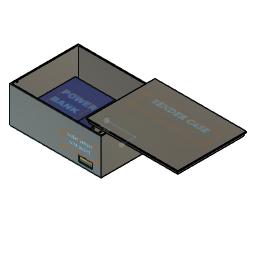
Sender case (Autodesk Fusion 360 design; units mm, degrees)
part number: 2025-07-08-07-24-11-456
Autodesk Fusion 360 part; units mm, degrees
sketch "Sketch1" plane through (0, 0, 0) normal (0, 0, 1) x (1, 0, 0)
  line L0 (80, -60) -> (-80, -60)
  line L1 (-80, -60) -> (-80, 60)
  line L2 (-80, 60) -> (80, 60)
  line L3 (80, 60) -> (80, -60)
  line L4 (80, -60) -> (-80, 60) construction
  line L5 (-80, -60) -> (80, 60) construction
  dimension "d1" = 160
  dimension "d2" = 120
  constraint horizontal L0
  constraint perpendicular L0 L1
  constraint parallel L0 L2
  constraint parallel L1 L3
  constraint coincident L4 origin
  constraint coincident L5 origin
  measures "d1" distance of L1.end L2.end
  measures "d2" distance of L0.end L1.end
extrude "Extrude1" add sketch "Sketch1" along normal blind 35 makes body 1
shell "Shell1" thickness 2 removed faces 1 at (26.6667, -20, 35) on bodies 1
sketch "Sketch2" plane through (0, 0, 35) normal (0, 0, 1) x (-1, 0, 0)
  line L0 (-78, -58) -> (-78, 58)
  line L1 (-78, 58) -> (78, 58)
  line L2 (78, 58) -> (78, -58)
  line L3 (78, -58) -> (-78, -58)
  line L4 (-80, -60) -> (80, -60)
  line L5 (80, -60) -> (80, 60)
  line L6 (80, 60) -> (-80, 60)
  line L7 (-80, 60) -> (-80, -60)
  line L8 (-80, -60) -> (80, -60)
  line L9 (80, -60) -> (80, 60)
extrude "Extrude2" add sketch "Sketch2" along normal blind 7 bodies 1
sketch "Sketch3" plane through (0, 0, 42) normal (0, 0, 1) x (-1, 0, 0)
  line L0 (78, 58) -> (78, -58)
  line L1 (78, -58) -> (-78, -58)
  line L2 (-78, -58) -> (-78, 58)
  line L3 (-78, 58) -> (78, 58)
  line L4 (80, -60) -> (80, 60)
  line L5 (80, 60) -> (-80, 60)
  line L6 (-80, 60) -> (-80, -60)
  line L7 (-80, -60) -> (80, -60)
extrude "Extrude3" add sketch "Sketch3" along normal blind 7 bodies 1
sketch "Sketch4" plane through (0, 0, 0) normal (0, 0, 1) x (1, 0, 0)
  line L0 (80, 60) -> (-80, 60)
  line L1 (-80, 60) -> (-80, -60)
  line L2 (-80, -60) -> (80, -60)
  line L3 (80, -60) -> (80, 60)
  line L4 (80, 60) -> (-80, -60) construction
  line L5 (-80, 60) -> (80, -60) construction
  dimension "d10" = 160
  dimension "d11" = 120
  constraint horizontal L0
  constraint perpendicular L0 L1
  constraint parallel L0 L2
  constraint parallel L1 L3
  constraint coincident L4 origin
  constraint coincident L5 origin
  measures "d10" distance of L1.end L2.end
  measures "d11" distance of L0.end L1.end
extrude "Extrude4" add sketch "Sketch4" along normal blind 7 separate body makes body 2
move_body "Move1" bodies 2 to x (1, 0, 0) y (0, 1, 0) z (0, 0, 1) at (0, 0, 40)
sketch "Sketch5" plane through (0, 0, 49) normal (0, 0, 1) x (-1, 0, 0)
  line L0 (-78, -58) -> (-78, 58)
  line L1 (-78, 58) -> (78, 58)
  line L2 (78, 58) -> (78, -58)
  line L3 (78, -58) -> (-78, -58)
  line L4 (-80, -60) -> (80, -60)
  line L5 (80, -60) -> (80, 60)
  line L6 (80, 60) -> (-80, 60)
  line L7 (-80, 60) -> (-80, -60)
extrude "Extrude5" add sketch "Sketch5" along normal blind 7 bodies 1
sketch "Sketch6" plane through (0, 0, 56) normal (0, 0, 1) x (-1, 0, 0)
  line L0 (78, 58) -> (78, -58)
  line L1 (78, -58) -> (-78, -58)
  line L2 (-78, -58) -> (-78, 58)
  line L3 (-78, 58) -> (78, 58)
  line L4 (-80, 60) -> (-80, -60)
  line L5 (-80, -60) -> (80, -60)
  line L6 (80, -60) -> (80, 60)
  line L7 (80, 60) -> (-80, 60)
  line L8 (-80, 60) -> (-80, -60)
  line L9 (80, 60) -> (-80, 60)
  line L10 (80, -60) -> (80, 60)
  line L11 (-80, -60) -> (80, -60)
extrude "Extrude6" add sketch "Sketch6" along normal blind 7 bodies 1
move_body "Move2" bodies 2 to x (1, 0, 0) y (0, 1, 0) z (0, 0, 1) at (-5.0948, 10.5251, 18.3046)
sketch "Sketch7" plane through (0, 0, 65.3046) normal (0, 0, 1) x (-1, 0, 0)
  line L0 (-74.9052, 49.4749) -> (-74.9052, -70.5251)
  line L1 (-74.9052, -70.5251) -> (85.0948, -70.5251)
  line L2 (85.0948, -70.5251) -> (85.0948, 49.4749)
  line L3 (85.0948, 49.4749) -> (-74.9052, 49.4749)
  line L4 (-74.9052, 49.4749) -> (-74.9052, -70.5251)
  line L5 (-74.9052, -70.5251) -> (85.0948, -70.5251)
  line L6 (85.0948, -70.5251) -> (85.0948, 49.4749)
  line L7 (85.0948, 49.4749) -> (-74.9052, 49.4749)
  line L8 (83.0948, -68.5251) -> (83.0948, 47.4749)
  line L9 (83.0948, 47.4749) -> (-72.9052, 47.4749)
  line L10 (-72.9052, 47.4749) -> (-72.9052, -68.5251)
  line L11 (-72.9052, -68.5251) -> (83.0948, -68.5251)
  dimension "d18" = -2
extrude "Extrude7" cut sketch "Sketch7" against normal blind 5 bodies 1 2
move_body "Move3" bodies 2 to x (1, 0, 0) y (0, 1, 0) z (0, 0, 1) at (0, -11, 0)
move_body "Move4" bodies 2 to x (1, 0, 0) y (0, -1, 0) z (0, 0, -1) at (140, -0.9498, 136.6091)
sketch "Sketch8" plane through (0, 0, 2) normal (0, 0, 1) x (-1, 0, 0)
  line L0 (-78, -58) -> (78, -58)
  line L1 (78, -58) -> (78, 58)
  line L2 (78, 58) -> (-78, 58)
  line L3 (-78, 58) -> (-78, -58)
  line L4 (181.9666, -46.9466) -> (111.9666, -46.9466)
  line L5 (111.9666, -46.9466) -> (111.9666, 53.0534)
  line L6 (111.9666, 53.0534) -> (181.9666, 53.0534)
  line L7 (181.9666, 53.0534) -> (181.9666, -46.9466)
  dimension "d21" = 70
  dimension "d22" = 100
  constraint horizontal L4
  constraint vertical L5
  constraint horizontal L6
  constraint vertical L7
  measures "d21" distance of L4.start L4.end
  measures "d22" distance of L4.start L6.end
extrude "Extrude8" add sketch "Sketch8" along normal blind 22 separate body contours L4 L5 L6 L7 makes body 3
move_body "Move5" bodies 3 to x (1, 0, 0) y (0, 1, 0) z (0, 0, 1) at (100, 0, 0)
move_body "Move6" bodies 3 to x (1, 0, 0) y (0, 1, 0) z (0, 0, 1) at (10, 0, 0)
other "Base Mesh Feature1"
other "Scale1"
other "Modify1"
other "Modify2"
other "Modify3"
other "Modify4"
other "Modify5"
other "Modify6"
other "Modify7"
other "Modify8"
other "Modify9"
other "Modify10"
other "Scale2"
other "Modify11"
other "Scale3"
other "Modify12"
other "Modify13"
sketch "Sketch9" plane through (0, 0, 24) normal (0, 0, 1) x (-1, 0, 0)
  line L0 (71.9666, 53.0534) -> (1.9666, 53.0534)
  line L1 (1.9666, 53.0534) -> (1.9666, -46.9466)
  line L2 (1.9666, -46.9466) -> (71.9666, -46.9466)
  line L3 (71.9666, -46.9466) -> (71.9666, 53.0534)
  line L4 (60, 30) -> (10, 30) construction
  line L5 (10, 30) -> (10, -20) construction
  line L6 (10, -20) -> (60, -20) construction
  line L7 (60, -20) -> (60, 30) construction
  line L8 (-25.6969, 10) -> (-40, 10) construction
  line L9 (-40, 10) -> (-40, 3.0534) construction
  line L10 (-40, 3.0534) -> (-25.6969, 3.0534) construction
  line L11 (-25.6969, 3.0534) -> (-25.6969, 10) construction
  line L12 (-70, 0, 55) -> (-200, 0, 55) construction
  line L13 (-200, 0, 55) -> (-200, -30, 55) construction
  line L14 (-200, -30, 55) -> (-70, -30, 55) construction
  line L15 (-70, -30, 55) -> (-70, 0, 55) construction
  dimension "d34" = 10
  dimension "d35" = 5
  dimension "d36" = 10
sketch "Sketch10" plane through (0, 0, 2) normal (0, 0, 1) x (-1, 0, 0)
  line L0 (-78, -58) -> (78, -58)
  line L1 (78, -58) -> (78, 58)
  line L2 (78, 58) -> (-78, 58)
  line L3 (-78, 58) -> (-78, -58)
  line L4 (0, -30) -> (-50, -30)
  line L5 (-50, -30) -> (-50, -5.6581)
  constraint horizontal L4
  constraint perpendicular L4 L5
sketch "Sketch11" plane through (0, -60, 0) normal (0, -1, 0) x (1, 0, 0)
  line L0 (-80, 0) -> (80, 0)
  line L1 (80, 0) -> (80, 63)
  line L2 (80, 63) -> (-80, 63)
  line L3 (-80, 63) -> (-80, 0)
  line L4 (40, 15) -> (65, 15)
  line L5 (65, 15) -> (65, 5)
  line L6 (65, 5) -> (40, 5)
  line L7 (40, 5) -> (40, 15)
  constraint horizontal L4
  constraint vertical L5
  constraint horizontal L6
  constraint vertical L7
extrude "Extrude9" cut sketch "Sketch11" against normal blind 2.2 contours L4 L5 L6 L7 bodies 1
other "Modify14"
sketch "Sketch12" plane through (0, -60, 0) normal (0, -1, 0) x (1, 0, 0)
  line L0 (65, 15) -> (65, 5)
  line L1 (65, 5) -> (40, 5)
  line L2 (40, 5) -> (40, 15)
  line L3 (40, 15) -> (65, 15)
  line L4 (-80, 0) -> (80, 0)
  line L5 (80, 0) -> (80, 63)
  line L6 (80, 63) -> (-80, 63)
  line L7 (-80, 63) -> (-80, 0)
  line L8 (10, 16.1796) -> (76.0063, 16.1796) construction
  line L9 (76.0063, 16.1796) -> (76.0063, 40) construction
  line L10 (76.0063, 40) -> (10, 40) construction
  line L11 (10, 40) -> (10, 16.1796) construction
  dimension "d39" = 5
